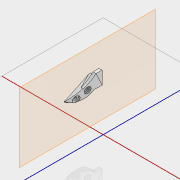
# Autodesk Inventor part: ЛЦМК.30000.10.00.04  Переходник
Saved by Autodesk Inventor 2021.2 (Build 252289000, 289)
## iProperties
Created: 2025-11-22
Part Number: ЛЦМК.30000.10.00.04  Переходник
Material: Типовые
Document SubType Name: Modeling
Designer: Захаров
Density: 1 g/cm^3
Appearance: По умолчанию
Author: Захаров
Autodesk Inventor part; units mm, degrees
ref_plane "YZ Plane" through (0, 0, 0) normal (1, 0, 0) x (0, 1, 0)
ref_plane "XZ Plane" through (0, 0, 0) normal (0, 1, 0) x (-1, 0, 0)
ref_plane "XY Plane" through (0, 0, 0) normal (0, 0, 1) x (1, 0, 0)
sketch "Эскиз1" plane through (0, 0, 0) normal (0, 0, 1) x (1, 0, 0)
  line L0 (-10, 17) -> (-7, 17) projected
  line L1 (-10, 4) -> (-10, 17) projected
  line L2 (-7, 4) -> (-10, 4) projected
  line L3 (-7, 17) -> (-7, 4) projected
  point P0 (0, 0)
ref_plane "РабПлоскость1" through (-13, -24, -6) normal (0, 0, -1) x (0, 1, 0)
extrude "Выдавливание1" add sketch "Эскиз1" against normal up to surface (6 mm away)
ref_plane "РабПлоскость2" through (-13, 2.5481, 2.5558) normal (1, 0, 0) x (0, 1, 0)
sketch "Эскиз3" plane through (-13, 2.5481, 2.5558) normal (1, 0, 0) x (0, 1, 0)
  line L0 (29.663, -39.7893) -> (-15.8657, 56.6115) projected
  line L1 (1.4519, -2.5558) -> (14.4519, -2.5558) projected
  circle A0 centre (3.4507, 4.8159) radius 1.5 projected
  circle A1 centre (-0.8198, 13.8581) radius 1.5 projected
  arc A2 (-0.157, 23.3504) -> (1.4519, -2.5558) centre (15.5518, 11.3229) ccw
  point P0 (-2.5481, -2.5558)
  point P1 (12.0781, -2.5558)
  constraints: 2 point on circle, 1 centre point, 1 point on line
ref_plane "РабПлоскость3" through (-7, 4, -6) normal (-1, 0, 0) x (0, 0, 1)
extrude "Выдавливание3" add sketch "Эскиз3" along normal up to surface (6 mm away)
fillet "Сопряжение1" radius 46.5 1 edges at (-8.5, 14.6263, 0)
fillet "Сопряжение2" radius 3.5 1 edges at (-10, 11.8609, 5.8552)
sketch "Эскиз4" plane through (-13, 2.3911, 25.9062) normal (0, 0.9042265, 0.4270533) x (1, 0, 0)
  line L0 (6, 15.6992) -> (6, 29.6638) projected
  arc A0 (0, 0) -> (6, 29.6638) centre (-70.3284, 29.6638) ccw
  line L1 (6, 15.6992) -> (6, 0) projected
  line L2 (0, 0) -> (6, 0) projected
  point P0 (13, 22.4039)
  constraints: 2 point on circle, 1 centre point, 1 tangent
extrude "Выдавливание4" cut sketch "Эскиз4" against normal mid plane 26.43
fillet "Сопряжение3" radius 1 2 edges at (-11.6601, -0.4302, 20.8113) (-8.2416, -0.4256, 6.9337)
sketch "Эскиз5" plane through (-7, 4.2958, -6) normal (1, 0, 0) x (0, 0, -1)
  spline S0 degree 2 poles (-13.3717, 3.2031) (-15.9697, 3.2031) (-14.6707, 0.9531) (-13.3717, -1.2969) (-12.0726, 0.9531) (-10.7736, 3.2031) (-13.3717, 3.2031) knots 0 0 0 0.333333 0.333333 0.666667 0.666667 1 1 1 weights 1 0.5 1 0.5 1 0.5 1 projected
  circle A0 centre (-13.3717, 1.7031) radius 3
  circle A1 centre (-13.3717, 1.7031) radius 1.5 projected
  circle A2 centre (-13.3717, 1.7031) radius 1.5 projected
  point P0 (-6, -4.2958)
  point P1 (-23.7703, -3.2081)
  point P2 (-23.7703, -3.2081)
  dimension "d12" = 6
  constraints: 1 centre point, 1 concentric, 2 other
  measures "d12" diameter of A0
extrude "Выдавливание5" cut sketch "Эскиз5" against normal blind 2.5
sketch "Эскиз6" plane through (-7, 4.2958, -6) normal (1, 0, 0) x (0, 0, -1)
  spline S0 degree 5 poles (-22.4139, -1.0675) (-22.6514, -1.0675) (-22.9007, -1.1148) (-23.1375, -1.2169) (-23.3436, -1.3662) (-23.6898, -1.735) (-23.8196, -1.9595) (-23.8969, -2.1971) (-23.9253, -2.4343) (-23.8896, -3.001) (-23.7727, -3.3225) (-23.5759, -3.6041) (-23.3009, -3.8301) (-22.7541, -4.0457) (-22.5155, -4.094) (-22.2614, -4.0923) (-22.0078, -4.0345) (-21.5399, -3.8135) (-21.3339, -3.6547) (-21.1707, -3.4593) (-21.0562, -3.2438) (-20.9113, -2.7958) (-20.887, -2.558) (-20.9077, -2.3258) (-20.969, -2.1067) (-21.2062, -1.6241) (-21.4192, -1.3791) (-21.6945, -1.1833) (-22.0433, -1.0675) (-22.4139, -1.0675) knots 0 0 0 0 0 0 0.11713 0.11713 0.11713 0.11713 0.247597 0.247597 0.247597 0.247597 0.442308 0.442308 0.442308 0.442308 0.563752 0.563752 0.563752 0.563752 0.684707 0.684707 0.684707 0.684707 0.816037 0.816037 0.816037 0.816037 1 1 1 1 1 1 projected
  circle A0 centre (-22.4139, -2.5675) radius 1.5 projected
  circle A1 centre (-22.4139, -2.5675) radius 3
  point P0 (-6, -4.2958)
  dimension "d16" = 6
  constraints: 1 centre point, 1 coincident, 2 other
  measures "d16" diameter of A1
extrude "Выдавливание6" cut sketch "Эскиз6" against normal blind 4
